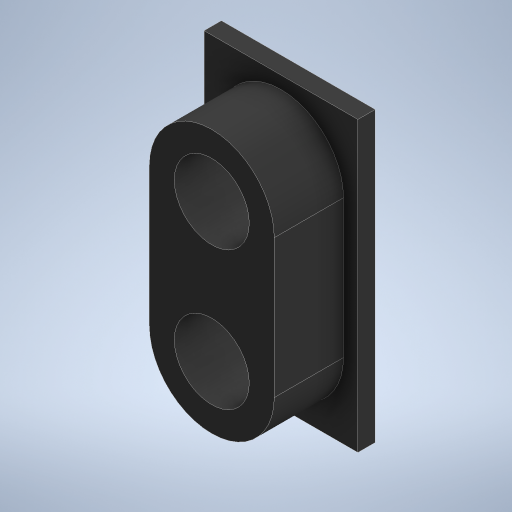
# Autodesk Inventor part: Double_Steckdose
Saved by Autodesk Inventor 2024 (Build 280153000, 153)
## iProperties
Created: 2026-05-31
Part Number: Double_Steckdose
Material: Gummi
Document SubType Name: Modeling
Designer: maxim
Density: 0.93 g/cm^3
Appearance: Gummi - Schwarz
Author: maxim
Autodesk Inventor part; units mm, degrees
ref_plane "YZ Plane" through (0, 0, 0) normal (1, 0, 0) x (0, 1, 0)
ref_plane "XZ Plane" through (0, 0, 0) normal (0, 1, 0) x (-1, 0, 0)
ref_plane "XY Plane" through (0, 0, 0) normal (0, 0, 1) x (1, 0, 0)
sketch "Skizze1" plane through (0, 0, 0) normal (0, 1, 0) x (-1, 0, 0)
  line L0 (0, 0) -> (80, 0)
  line L1 (80, 0) -> (80, -150)
  line L2 (80, -150) -> (0, -150)
  line L3 (0, -150) -> (0, 0)
  dimension "d0" = 80
  dimension "d1" = 150
  constraints: 8 end point, 2 parallel, 1 horizontal, 1 perpendicular
  measures "d0" distance of L1.end L2.end
  measures "d1" distance of L0.end L1.end
extrude "Extrusion1" add sketch "Skizze1" along normal blind 10
sketch "Skizze2" plane through (0, 10, 0) normal (0, 1, 0) x (1, 0, 0)
  circle A0 centre (-40, 39) radius 19.5
  line L0 (-80, 0) -> (0, 0) projected
  line L1 (0, 150) -> (-80, 150) projected
  line L2 (-80, 150) -> (-80, 0) projected
  line L3 (-80, 75) -> (0, 75)
  circle A1 centre (-40, 111) radius 19.5
  dimension "d4" = 39
  dimension "d5" = 72
  constraints: 2 centre point, 2 end point, 1 horizontal, 1 midpoint, 1 symmetric about line, 1 other
  measures "d4" diameter of A0
  measures "d5" diameter of A0.centre L3
extrude "Extrusion2" cut sketch "Skizze2" against normal blind 10
sketch "Skizze3" plane through (0, 0, 0) normal (0, -1, 0) x (1, 0, 0)
  circle A0 centre (-40, -111) radius 19.5 projected
  circle A1 centre (-40, -39) radius 19.5 projected
  line L0 (-40, -111) -> (-40, -39) construction
  line L1 (-7.5, -111) -> (-7.5, -39)
  line L2 (-72.5, -39) -> (-72.5, -111)
  arc A2 (-72.5, -111) -> (-7.5, -111) centre (-40, -111) ccw
  arc A3 (-7.5, -39) -> (-72.5, -39) centre (-40, -39) ccw
  point P0 (0, 0)
  point P1 (-40, -75)
  dimension "d8" = 65
  constraints: 8 end point, 4 point on circle, 4 tangent, 2 centre point, 1 midpoint, 1 parallel, 1 vertical
  measures "d8" distance between parallel lines of L1 L2
extrude "Extrusion3" add sketch "Skizze3" along normal blind 36
chamfer "Fasen1" distance 1 angle 45 4 edges at (-80, 10, -75) (-40, 10, -150) (0, 10, -75) (-40, 10, 0)
